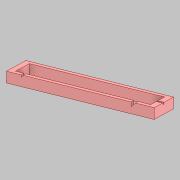
# Autodesk Inventor part: B1-X
Saved by Autodesk Inventor 2018.1 (Build 221171000, 171)
## iProperties
Created: 2018-06-22
Part Number: B1-X
Material: Všeobecné
Document SubType Name: Modeling
Designer: PS
Density: 1 g/cm^3
Appearance: Výchozí
Author: PS
Autodesk Inventor part; units mm, degrees
ref_plane "YZ Plane" through (0, 0, 0) normal (1, 0, 0) x (0, 1, 0)
ref_plane "XZ Plane" through (0, 0, 0) normal (0, 1, 0) x (-1, 0, 0)
ref_plane "Pracovní rovina1" through (0, 0, 0) normal (0, 0, 1) x (1, 0, 0)
sketch "Náčrt1" plane through (0, 0, 0) normal (0, 0, 1) x (1, 0, 0)
  line L0 (0, 0) -> (1400, 0)
  line L1 (1400, 0) -> (1400, 7000)
  line L2 (1400, 7000) -> (0, 7000)
  line L3 (0, 7000) -> (0, 0)
  line L4 (200, 6700) -> (1200, 6700)
  line L5 (1200, 6700) -> (1200, 300)
  line L6 (1200, 300) -> (200, 300)
  line L7 (200, 300) -> (200, 6700)
  dimension "d13" = 7000
  dimension "d14" = 1000
  dimension "d15" = 300
  dimension "d16" = 300
  dimension "d17" = 200
  dimension "d18" = 200
  constraints: 16 end point, 4 parallel, 2 horizontal, 2 perpendicular
  measures "d13" distance between parallel lines of L0 L2
  measures "d14" distance of L5.end L6.end
  measures "d15" distance between parallel lines of L4 L2
  measures "d16" distance between parallel lines of L0 L6
  measures "d17" distance between parallel lines of L3 L7
  measures "d18" distance between parallel lines of L1 L5
extrude "Vysunutí1" add sketch "Náčrt1" along normal blind 500
sketch "Náčrt2" plane through (0, 6700, 0) normal (-1, 0, 0) x (0, 1, 0)
  line L0 (-400, -500) -> (-400, -400)
  line L1 (-400, -400) -> (-500, -500)
  line L2 (-500, -500) -> (-400, -500)
  line L3 (300, -500) -> (-6700, -500) projected
  line L4 (300, 0) -> (300, -500) projected
  line L5 (-5606.35, -500) -> (-5606.35, -300)
  line L6 (-5606.35, -300) -> (-5806.35, -500)
  line L7 (-5606.35, -500) -> (-5806.35, -500)
  point P0 (-6700, 0)
  dimension "d7" = 100
  dimension "d19" = 700
  dimension "d24" = 45
  dimension "d25" = 5206.35
  dimension "d26" = 200
  constraints: 12 end point, 2 collinear, 2 perpendicular, 2 point on line, 2 vertical
  measures "d7" distance of L0.start L0.end
  measures "d19" distance between parallel lines of L4 L0
  measures "d24" angle of L0 L1
  measures "d25" distance between parallel lines of L0 L5
  measures "d26" distance of L5.start L5.end
extrude "Vysunutí2" cut sketch "Náčrt2" against normal blind 293.5
sketch "Náčrt3" plane through (0, 0, 0) normal (0, -1, 0) x (1, 0, 0)
  line L0 (0, 500) -> (1400, 500) projected
  line L1 (600, 500) -> (700, 400)
  line L2 (700, 500) -> (700, 400)
  point P0 (0, 0)
  dimension "d20" = 45
  dimension "d21" = 100
  constraints: 4 end point, 1 midpoint, 1 perpendicular, 1 point on line
  measures "d20" angle of L1 L2
  measures "d21" distance of L2.start L1.end
extrude "Vysunutí3" cut sketch "Náčrt3" against normal blind 358
equation "\"d16\" = d15"
equation "\"d18\" = d17"
